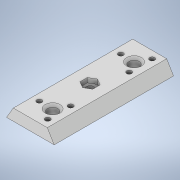
# Autodesk Inventor part: Motor_holder
Saved by Autodesk Inventor 2021 (Build 250183000, 183)
## iProperties
Created: 2024-05-11
Part Number: Motor_holder
Material: Generic
Document SubType Name: Modeling
Designer: Lukas
Density: 1 g/cm^3
Appearance: Default
Author: Lukas
Autodesk Inventor part; units mm, degrees
ref_plane "YZ Plane" through (0, 0, 0) normal (1, 0, 0) x (0, 1, 0)
ref_plane "XZ Plane" through (0, 0, 0) normal (0, 1, 0) x (-1, 0, 0)
ref_plane "XY Plane" through (0, 0, 0) normal (0, 0, 1) x (1, 0, 0)
sketch "Sketch5" plane through (0, 0, 0) normal (0, 0, 1) x (1, 0, 0)
  line L0 (-7.4, 2.5) -> (7.4, 2.5)
  line L1 (7.4, 2.5) -> (10.4, -2.5)
  line L2 (10.4, -2.5) -> (-10.4, -2.5)
  line L3 (-10.4, -2.5) -> (-7.4, 2.5)
  point P0 (0, 0)
  point P1 (0, 2.5)
  point P2 (-8.9, 0)
  dimension "d38" = 14.8
  dimension "d39" = 20.8
  dimension "d40" = 5
  constraints: 8 end point, 2 midpoint, 1 equal length, 1 horizontal, 1 horizontal alignment, 1 parallel, 1 vertical alignment
  measures "d38" distance of L0.start L0.end
  measures "d39" distance of L1.end L2.end
  measures "d40" distance between parallel lines of L2 L0
extrude "Extrusion5" add sketch "Sketch5" along normal mid plane 52
sketch "Sketch1" plane through (0, 2.5, -26) normal (0, 1, 0) x (1, 0, 0)
  circle A0 centre (1.4439, -43.75) radius 2.25
  circle A1 centre (-4.3301, -43.75) radius 1.1
  circle A2 centre (4.3301, -38.75) radius 1.1
  circle A3 centre (4.3301, -48.75) radius 1.1
  circle A4 centre (1.4439, -8.25) radius 2.25
  circle A5 centre (-4.3301, -8.25) radius 1.1
  circle A6 centre (4.3301, -3.25) radius 1.1
  circle A7 centre (4.3301, -13.25) radius 1.1
  circle A8 centre (0, -26) radius 1.6
  line L0 (7.4, 0) -> (7.4, -52) projected
  line L1 (-7.4, 0) -> (-7.4, -52) projected
  dimension "d0" = 10
  dimension "d1" = 10
  dimension "d2" = 10
  dimension "d3" = 5
  dimension "d4" = 5.774
  dimension "d11" = 2.2
  dimension "d12" = 4.5
  dimension "d43" = 10
  dimension "d44" = 10
  dimension "d45" = 10
  dimension "d46" = 5
  dimension "d47" = 5.774
  dimension "d48" = 2.2
  dimension "d49" = 4.5
  dimension "d51" = 35.5
  dimension "d60" = 3.2
  dimension "d65" = 3.0699
  dimension "d66" = 3.0699
  dimension "d67" = 17.75
  constraints: 9 centre point, 4 equal radius, 3 coincident, 3 vertical alignment
  measures "d0" distance of A3.centre A2.centre
  measures "d1" distance of A1.centre A3.centre
  measures "d2" distance of A1.centre A2.centre
  measures "d3" vertical distance of A2.centre A0.centre
  measures "d4" distance of A1.centre A0.centre
  measures "d11" diameter of A2
  measures "d12" diameter of A0
  measures "d43" distance of A7.centre A6.centre
  measures "d44" distance of A5.centre A7.centre
  measures "d45" distance of A5.centre A6.centre
  measures "d46" vertical distance of A6.centre A4.centre
  measures "d47" distance of A5.centre A4.centre
  measures "d48" diameter of A6
  measures "d49" diameter of A4
  measures "d51" distance of point (1.444, -8.25) point (1.444, -43.75)
  measures "d60" diameter of A8
  measures "d65" distance from line of L0 A7.centre
  measures "d66" distance from line of L1 A5.centre
  measures "d67" vertical distance of point (0, -26) point (1.444, -43.75)
extrude "Extrusion6" cut sketch "Sketch1" against normal through all
sketch "Sketch6" plane through (-10.4, -2.5, 26) normal (0, -1, 0) x (1, 0, 0)
  circle A0 centre (6.0699, -8.25) radius 1.1 projected
  circle A1 centre (14.7301, -48.75) radius 1.1 projected
  circle A2 centre (6.0699, -43.75) radius 1.1 projected
  circle A3 centre (11.8439, -8.25) radius 2.25 projected
  circle A4 centre (14.7301, -13.25) radius 1.1 projected
  circle A5 centre (14.7301, -38.75) radius 1.1 projected
  circle A6 centre (11.8439, -43.75) radius 2.25 projected
  circle A7 centre (14.7301, -3.25) radius 1.1 projected
  line L0 (20.8, -52) -> (20.8, 0) projected
  line L1 (0, 0) -> (20.8, 0) projected
  line L2 (0, 0) -> (0, -52) projected
  line L3 (20.8, -52) -> (0, -52) projected
  circle A8 centre (14.7301, -13.25) radius 2.25
  circle A9 centre (14.7301, -3.25) radius 2.25
  circle A10 centre (6.0699, -8.25) radius 1.1 projected
  circle A11 centre (6.0699, -8.25) radius 2.25
  circle A12 centre (14.7301, -38.75) radius 1.1 projected
  circle A13 centre (14.7301, -38.75) radius 2.25
  circle A14 centre (14.7301, -48.75) radius 2.25
  circle A15 centre (6.0699, -43.75) radius 2.25
  point P0 (10.4, -26)
  dimension "d54" = 4.5
  constraints: 6 centre point, 6 coincident, 5 equal radius
  measures "d54" diameter of A8
extrude "Extrusion7" cut sketch "Sketch6" against normal blind 2 contours A8 | A9 | A11 | A13 | A14 | A15
sketch "Sketch7" plane through (-7.4, 2.5, 26) normal (0, 1, 0) x (1, 0, 0)
  circle A0 centre (7.4, 26) radius 1.6 projected
  circle A1 centre (7.4, 26) radius 1.6 projected
  line L0 (7.4, 29.2332) -> (10.2, 27.6166)
  line L1 (10.2, 27.6166) -> (10.2, 24.3834)
  line L2 (10.2, 24.3834) -> (7.4, 22.7668)
  line L3 (7.4, 22.7668) -> (4.6, 24.3834)
  line L4 (4.6, 24.3834) -> (4.6, 27.6166)
  line L5 (4.6, 27.6166) -> (7.4, 29.2332)
  dimension "d64" = 5.6
  constraints: 12 end point, 1 coincident, 1 vertical alignment, 13 other
  measures "d64" distance between parallel lines of L0 L3
extrude "Extrusion8" cut sketch "Sketch7" against normal blind 2
chamfer "Chamfer2" distance 1 angle 45 2 edges at (-0.8061, 2.5, 17.75) (-0.8061, 2.5, -17.75)
sketch "Sketch8" plane through (-7.4, 2.5, 26) normal (0, 1, 0) x (1, 0, 0)
  line L0 (-5.6, 13.5) -> (-1.6, 17)
  line L1 (-1.6, 17) -> (-1.6, 35)
  line L2 (-1.6, 35) -> (-5.6, 38.5)
  line L3 (-5.6, 38.5) -> (-5.6, 13.5)
  point P0 (7.4, 26)
  point P1 (-1.6, 26)
  point P2 (-5.6, 26)
  dimension "d68" = 9
  dimension "d70" = 4
  dimension "d71" = 18
  dimension "d72" = 25
  constraints: 8 end point, 2 horizontal alignment, 2 midpoint, 1 equal length, 1 parallel, 1 vertical
  measures "d68" distance from line of point (7.4, 26) L1
  measures "d70" distance between parallel lines of L3 L1
  measures "d71" distance of L0.end L1.end
  measures "d72" distance of L2.end L0.start
extrude "Extrusion9" cut sketch "Sketch8" against normal through all
equation "\"d1\" = d0"
equation "\"d2\" = d0"
equation "\"d3\" = 0.5 * d0"
equation "\"d44\" = d43"
equation "\"d45\" = d43"
equation "\"d46\" = 0.5 * d43"
equation "\"d66\" = d65"
equation "\"d67\" = 0.5 * d51"
body "Solid1"
body "Solid2"
